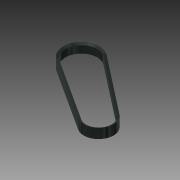
# Autodesk Inventor part: 砂轮皮带
Saved by Autodesk Inventor 2015 (Build 190159000, 159)
## iProperties
Created: 2017-05-24
Part Number: 砂轮皮带
Material: 常规
Document SubType Name: Modeling
Designer: Administrator
Density: 1 g/cm^3
Appearance: 铁灰色 - 抛光
Author: Administrator
Autodesk Inventor part; units mm, degrees
ref_plane "YZ Plane" through (0, 0, 0) normal (1, 0, 0) x (0, 1, 0)
ref_plane "XZ Plane" through (0, 0, 0) normal (0, 1, 0) x (-1, 0, 0)
ref_plane "XY Plane" through (0, 0, 0) normal (0, 0, 1) x (1, 0, 0)
sketch "草图1" plane through (0, 0, 0) normal (0, 0, 1) x (1, 0, 0)
  circle A0 centre (-95, 67.5) radius 25
  circle A1 centre (0, 0) radius 20
  line L0 (-79.6588, 87.2395) -> (12.273, 15.7916)
  line L1 (-108.5925, 46.518) -> (-10.874, -16.7856)
  line L2 (-77.511, 90.003) -> (14.4207, 18.5551)
  line L3 (-110.4954, 43.5805) -> (-12.7769, -19.7231)
  arc A2 (-77.511, 90.003) -> (-110.4954, 43.5805) centre (-95, 67.5) ccw
  arc A3 (-12.7769, -19.7231) -> (14.4207, 18.5551) centre (0, 0) ccw
  dimension "d0" = 50
  dimension "d1" = 40
  dimension "d2" = 95
  dimension "d3" = 67.5
  dimension "d4" = 3.5
  dimension "d5" = 3.5
  constraints: 8 end point, 8 point on circle, 6 tangent, 4 centre point, 2 concentric, 2 parallel, 1 coincident
  measures "d0" diameter of A0
  measures "d1" diameter of A1
  measures "d2" horizontal distance of A1.centre A0.centre
  measures "d3" vertical distance of A0.centre A1.centre
  measures "d4" distance between parallel lines of L0 L2
  measures "d5" distance between parallel lines of L1 L3
extrude "拉伸1" add sketch "草图1" along normal blind 15.423
chamfer "倒角1" distance 3.5 distance2 2.021 4 edges at (16.3036, -11.5841, 15.423) (-59.7332, 14.8662, 15.423) (-115.3795, 81.9802, 15.423) (-33.6929, 51.5155, 15.423) measured on face at (-16.9391, 41.4499, 15.423)
chamfer "倒角2" distance 3.5 distance2 2.021 4 edges at (-59.7332, 14.8662, 0) (16.3036, -11.5841, 0) (-33.6929, 51.5155, 0) (-115.3795, 81.9802, 0) measured on face at (-16.9391, 41.4499, 0)
